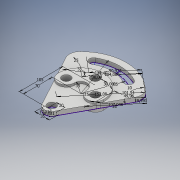
# Autodesk Inventor part: lab2_1_2
Saved by Autodesk Inventor 2018 (Build 220112000, 112)
## iProperties
Created: 2020-04-08
Part Number: lab2_1_2
Material: Типовые
Document SubType Name: Modeling
Designer: Antony
Density: 1 g/cm^3
Appearance: По умолчанию
Author: Antony
Autodesk Inventor part; units mm, degrees
ref_plane "YZ Plane" through (0, 0, 0) normal (1, 0, 0) x (0, 1, 0)
ref_plane "XZ Plane" through (0, 0, 0) normal (0, 1, 0) x (-1, 0, 0)
ref_plane "XY Plane" through (0, 0, 0) normal (0, 0, 1) x (1, 0, 0)
sketch "Эскиз1" plane through (0, 0, 0) normal (0, 0, 1) x (1, 0, 0)
  circle A0 centre (0, 0) radius 17.5
  circle A1 centre (0, 0) radius 10
  line L0 (0, 0) -> (0, 70)
  arc A2 (35, 70) -> (-35, 70) centre (0, 70) ccw
  arc A3 (55, 70) -> (-55, 70) centre (0, 70) ccw
  arc A4 (15, 70) -> (-15, 70) centre (0, 70) ccw
  arc A5 (-55, 70) -> (-15, 70) centre (-35, 70) ccw
  arc A6 (15, 70) -> (55, 70) centre (35, 70) ccw
  circle A7 centre (-35, 70) radius 10
  circle A8 centre (0, 105) radius 10
  circle A9 centre (35, 70) radius 10
  line L1 (-35, 70) -> (-35, 50)
  line L2 (-35, 50) -> (-35, 44.4464)
  line L3 (35, 70) -> (35, 50)
  line L4 (35, 50) -> (35, 44.4464)
  arc A10 (55, 165.2628) -> (0, 180) centre (0, 70) ccw
  line L5 (0, 70) -> (55, 165.2628) construction
  line L6 (0, 70) -> (0, 180) construction
  arc A11 (0, 180) -> (-55, 165.2628) centre (0, 70) ccw
  line L7 (0, 70) -> (-55, 165.2628) construction
  line L8 (0, 70) -> (0, 180) construction
  arc A12 (42.5, 143.6122) -> (-42.5, 143.6122) centre (0, 70) ccw
  arc A13 (37.5, 134.9519) -> (47.5, 152.2724) centre (42.5, 143.6122) ccw
  arc A14 (-47.5, 152.2724) -> (-37.5, 134.9519) centre (-42.5, 143.6122) ccw
  arc A15 (47.5, 152.2724) -> (-47.5, 152.2724) centre (0, 70) ccw
  arc A16 (37.5, 134.9519) -> (-37.5, 134.9519) centre (0, 70) ccw
  line L9 (0, 0) -> (-17.5, 0)
  line L10 (0, 0) -> (17.5, 0)
  line L11 (0, 0) -> (-10, 0)
  line L12 (0, 0) -> (10, 0)
  line L13 (0, 70) -> (0, 180)
  arc A17 (-55, 165.2628) -> (-70.7066, 154.2649) centre (0, 70) ccw
  line L14 (0, 70) -> (-55, 165.2628) construction
  line L15 (0, 70) -> (55, 165.2628)
  arc A18 (70.764, 154.2167) -> (55, 165.2628) centre (0, 70) ccw
  line L16 (-16.7681, -5.0081) -> (-83.5023, 117.8971)
  arc A19 (-70.7066, 154.2649) -> (-77.7825, 147.781) centre (0, 70) ccw
  arc A20 (-77.7825, 147.781) -> (-83.5023, 117.8971) centre (-61.1578, 129.1097) ccw
  line L17 (16.7749, -4.9852) -> (83.4973, 117.9265)
  line L18 (70.764, 154.2167) -> (80.7777, 145.8026)
  arc A21 (83.4973, 117.9265) -> (80.7777, 145.8026) centre (61.5259, 129.8537) ccw
  dimension "d15" = 70
  dimension "d17" = 105
  dimension "d19" = 30
  dimension "d20" = 30
  dimension "d23" = 10
  dimension "d28" = 35
  dimension "d29" = 20
  dimension "d30" = 20
  dimension "d31" = 15
  dimension "d32" = 35
  dimension "d33" = 85
  dimension "d34" = 110
  dimension "d35" = 55
  dimension "d55" = 25
  dimension "d110" = 19.5925
  dimension "d111" = 107.0482
  dimension "d112" = 152.0798
  dimension "d113" = 104.0886
  dimension "d114" = 90.9725
  dimension "d115" = 101.544
  dimension "d116" = 49.961
  dimension "d117" = 21.46
  dimension "d119" = 17.1211
  dimension "d120" = 17.1257
  constraints: 43 point on circle, 38 end point, 22 centre point, 17 coincident, 9 point on line, 8 tangent, 4 equal radius, 3 vertical, 2 horizontal, 1 collinear, 1 equal length
  measures "d15" distance of L0.end point (0, 0)
  measures "d17" distance of point (0, 0) A8.centre
  measures "d19" angle of L5 L6
  measures "d20" angle of L8 L7
  measures "d23" radius of A13
  measures "d28" distance of L10.end L9.end
  measures "d29" distance of L12.end L11.end
  measures "d30" diameter of A9
  measures "d31" radius of A4
  measures "d32" radius of A2
  measures "d33" radius of A12
  measures "d34" radius of A11
  measures "d35" radius of A3
  measures "d55" radius of A20
  measures "d110" distance from line of L17.end L18
  measures "d111" distance from line of L4.end L18
  measures "d112" distance from line of L2.end L18
  measures "d113" distance from line of A20.centre L18
  measures "d114" distance from line of A17.end L18
  measures "d115" angle of L17 L18
  measures "d116" angle of L3 L18
  measures "d117" angle of L16 L18
  measures "d119" distance from line of point (0, 0) L17
  measures "d120" distance from line of point (0, 0) L16
extrude "Выдавливание1" add sketch "Эскиз1" along normal blind 10 contours L9 A1 L10 A0 | A0 L16 A5 A4 L13 L0 | A0 L0 A1 L9 | L0 L15 A4 A6 L17 A0 | A0 L10 A1 L0 | L16 A5 A3 L13 A8 A2 A7 L1 | L13 A4 L15 | A6 L3 A9 A2 L15 A3 L17 | L16 A20 A19 A17 A11 L13 A15 A14 A16 A3 A5 | L1 A7 A2 A8 L13 A4 A5 | L13 A8 A2 L15 A4 | L15 A2 A9 L3 A6 A4 | A6 A3 L15 A13 A18 L18 A21 L17 | A2 A8 L13 A3 L15 | L13 A16 L15 A3 | A15 L13 A10 L15
extrude "Выдавливание2" add sketch "Эскиз1" along normal blind 15 and the other way blind 7.5 contours L16 A5 A3 L13 A8 A2 A7 L1 | A5 L16 | L17 A6 | A6 L3 A9 A2 L15 A3 L17 | L1 A7 A2 A8 L13 A4 A5 | L13 A8 A2 L15 A4 | L15 A2 A9 L3 A6 A4 | A2 A8 L13 A3 L15
